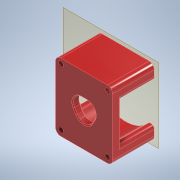
# Autodesk Inventor part: ESP32ParasiteMicroscope_top_v0
Saved by Autodesk Inventor 2022 (Build 260153000, 153)
## iProperties
Created: 2022-02-02
Part Number: ESP32ParasiteMicroscope_top_v0
Material: Generisch
Document SubType Name: Modeling
Designer: diederichbenedict
Density: 1 g/cm^3
Appearance: Rot
Author: diederichbenedict
Autodesk Inventor part; units mm, degrees
ref_plane "YZ Plane" through (0, 0, 0) normal (1, 0, 0) x (0, 1, 0)
ref_plane "XZ Plane" through (0, 0, 0) normal (0, 1, 0) x (-1, 0, 0)
ref_plane "XY Plane" through (0, 0, 0) normal (0, 0, 1) x (1, 0, 0)
ref_plane "Work Plane2" through (-11.0077, 0, -6) normal (0, 0, 1) x (1, 0, 0)
sketch "Sketch5" plane through (-11.0077, 0, -6) normal (0, 0, 1) x (1, 0, 0)
  circle A0 centre (-4.8724, 16.4874) radius 1.45 projected
  circle A1 centre (22, 16.4874) radius 1.45 projected
  circle A2 centre (22, -16.4874) radius 1.45 projected
  circle A3 centre (-4.8724, -16.4874) radius 1.45 projected
  circle A4 centre (8.5638, 0) radius 6 projected
  circle A5 centre (-4.8724, 16.4874) radius 1.45 projected
  circle A6 centre (22, -16.4874) radius 1.45 projected
  circle A7 centre (-4.8724, -16.4874) radius 1.45 projected
  circle A8 centre (22, 16.4874) radius 1.45 projected
  arc A9 (-25, -16.4874) -> (-22, -19.4874) centre (-22, -16.4874) ccw projected
  line L0 (-22, -19.4874) -> (22, -19.4874) projected
  arc A10 (22, -19.4874) -> (25, -16.4874) centre (22, -16.4874) ccw projected
  line L1 (25, -16.4874) -> (25, 16.4874) projected
  arc A11 (25, 16.4874) -> (22, 19.4874) centre (22, 16.4874) ccw projected
  line L2 (22, 19.4874) -> (-22, 19.4874) projected
  arc A12 (-22, 19.4874) -> (-25, 16.4874) centre (-22, 16.4874) ccw projected
  line L3 (-25, 16.4874) -> (-25, -16.4874) projected
  line L4 (12.6638, -4.1) -> (4.4638, -4.1) projected
  line L5 (4.4638, -4.1) -> (4.4638, 4.1) projected
  line L6 (4.4638, 4.1) -> (12.6638, 4.1) projected
  line L7 (12.6638, 4.1) -> (12.6638, -4.1) projected
  circle A13 centre (-22, -16.4874) radius 1.4 projected
  circle A14 centre (-22, 16.4874) radius 1.15 projected
  line L8 (-4.8724, -19.4874) -> (22, -19.4874)
  line L9 (25, -16.4874) -> (25, 16.4874)
  line L10 (22, 19.4874) -> (-4.8724, 19.4874)
  line L11 (-7.8724, 16.4874) -> (-7.8724, -16.4874)
  line L12 (-7.8724, -19.4874) -> (25, 19.4874) construction
  line L13 (25, -19.4874) -> (-7.8724, 19.4874) construction
  arc A15 (-4.8724, 19.4874) -> (-7.8724, 16.4874) centre (-4.8724, 16.4874) ccw
  arc A16 (25, 16.4874) -> (22, 19.4874) centre (22, 16.4874) ccw
  arc A17 (22, -19.4874) -> (25, -16.4874) centre (22, -16.4874) ccw
  arc A18 (-7.8724, -16.4874) -> (-4.8724, -19.4874) centre (-4.8724, -16.4874) ccw
  circle A19 centre (8.5638, 0) radius 17.5
  point P0 (11.0077, 0)
  point P1 (-7.8724, 6.0085)
  point P2 (-7.8724, -6.0085)
  point P3 (25, 6.0085)
  point P4 (25, -6.0085)
  point P5 (25, -6.0085)
  point P6 (-4.8724, -19.4874)
  point P7 (25, 6.0085)
  point P8 (-4.8724, 19.4874)
  dimension "d17" = 3
  dimension "d18" = 35
  constraints: 12 end point, 12 point on circle, 12 point on line, 8 tangent, 5 centre point, 3 equal radius, 2 midpoint, 2 parallel, 1 coincident, 1 horizontal, 1 perpendicular
  measures "d17" radius of A15
  measures "d18" diameter of A19
extrude "Extrusion4" add sketch "Sketch5" along normal blind 20 contours A18 L11 A19 L1 A10 L0 | L2 A11 L1 A19 L11 A15
sketch "Sketch6" plane through (-11.0077, 0, 14) normal (0, 0, 1) x (1, 0, 0)
  line L0 (25, 6.0085) -> (25, 16.4874) projected
  arc A0 (25, 16.4874) -> (22, 19.4874) centre (22, 16.4874) ccw projected
  line L1 (22, 19.4874) -> (-4.8724, 19.4874) projected
  arc A1 (-4.8724, 19.4874) -> (-7.8724, 16.4874) centre (-4.8724, 16.4874) ccw projected
  line L2 (-7.8724, 16.4874) -> (-7.8724, 6.0085) projected
  arc A2 (25, 6.0085) -> (-7.8724, 6.0085) centre (8.5638, 0) ccw projected
  circle A3 centre (-4.8724, 16.4874) radius 1.45 projected
  circle A4 centre (22, 16.4874) radius 1.45 projected
  line L3 (-7.8724, -6.0085) -> (-7.8724, -16.4874) projected
  arc A5 (-7.8724, -16.4874) -> (-4.8724, -19.4874) centre (-4.8724, -16.4874) ccw projected
  line L4 (-4.8724, -19.4874) -> (22, -19.4874) projected
  arc A6 (22, -19.4874) -> (25, -16.4874) centre (22, -16.4874) ccw projected
  line L5 (25, -16.4874) -> (25, -6.0085) projected
  arc A7 (-7.8724, -6.0085) -> (25, -6.0085) centre (8.5638, 0) ccw projected
  circle A8 centre (-4.8724, -16.4874) radius 1.45 projected
  circle A9 centre (22, -16.4874) radius 1.45 projected
  arc A10 (25, 6.0085) -> (-7.8724, 6.0085) centre (8.5638, 0) ccw projected
  line L6 (25, 6.0085) -> (25, -6.0085)
  arc A11 (-7.8724, -6.0085) -> (25, -6.0085) centre (8.5638, 0) ccw projected
  line L7 (-7.8724, 6.0085) -> (-7.8724, -6.0085)
  circle A12 centre (8.5638, 0) radius 6 construction
  circle A13 centre (8.5638, 0) radius 5.9 construction
  line L8 (7.005, 5.9) -> (10.1227, 5.9)
  line L9 (14.4528, -1.6) -> (12.8939, -4.3)
  line L10 (4.2337, -4.3) -> (2.6749, -1.6)
  arc A14 (7.005, 5.9) -> (2.6749, -1.6) centre (7.005, 0.9) ccw
  arc A15 (14.4528, -1.6) -> (10.1227, 5.9) centre (10.1227, 0.9) ccw
  arc A16 (4.2337, -4.3) -> (12.8939, -4.3) centre (8.5638, -1.8) ccw
  point P0 (11.0077, 0)
  point P1 (-1.6553, 5.9)
  point P2 (18.7829, 5.9)
  point P3 (8.5638, -11.8)
  dimension "d24" = 11.8
  dimension "d28" = 5
  constraints: 10 end point, 7 point on circle, 7 point on line, 7 tangent, 4 centre point, 2 coincident, 2 collinear, 2 equal radius, 1 parallel, 7 other
  measures "d24" diameter of A13
  measures "d28" radius of A14
extrude "Extrusion5" add sketch "Sketch6" along normal blind 4
fillet "Fillet1" radius 2 4 edges at (-18.8801, 6.0085, 4) (-18.8801, -6.0085, 4) (13.9923, 6.0085, 4) (13.9923, -6.0085, 4)
chamfer "Chamfer1" distance 0.5 angle 45 12 edges at (-8.3329, 3.4, 18) (-2.4439, 5.9, 18) (3.4451, 3.4, 18) (2.6656, -2.95, 18) (-2.4439, -6.8, 18) (-7.5535, -2.95, 18) (-8.3329, 3.4, 14) (-2.4439, 5.9, 14) (3.4451, 3.4, 14) (2.6656, -2.95, 14) (-2.4439, -6.8, 14) (-7.5535, -2.95, 14)
body "Solid2"
